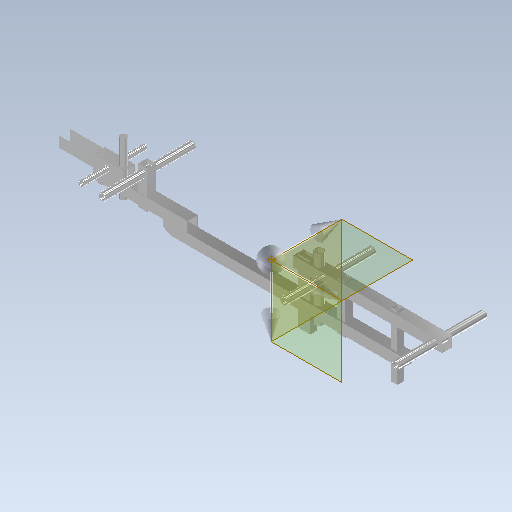
# Autodesk Inventor part: skeleton1
Saved by Autodesk Inventor 2020 (Build 240168000, 168)
## iProperties
Created: 2016-11-12
Part Number: skeleton1
Material: Aluminum 6061
Document SubType Name: Modeling
Designer: jous
Density: 2.7 g/cm^3
Appearance: Aluminum - Flat
Mass: 2970.51 g
Surface Area: 10814.6 cm^2
Volume: 1100.19 cm^3
Author: jous
Autodesk Inventor part; units mm, degrees
ref_plane "YZ Plane" through (0, 0, 0) normal (1, 0, 0) x (0, 1, 0)
ref_plane "XZ Plane" through (0, 0, 0) normal (0, 1, 0) x (-1, 0, 0)
ref_plane "XY Plane" through (0, 0, 0) normal (0, 0, 1) x (1, 0, 0)
sketch "cross" plane through (0, 0, 0) normal (0, 0, 1) x (1, 0, 0)
  line L0 (-20, -20) -> (20, -20)
  line L1 (20, -20) -> (20, 20)
  line L2 (20, 20) -> (-20, 20)
  line L3 (-20, 20) -> (-20, -20)
  line L4 (-20, -20) -> (20, 20) construction
  line L5 (20, -20) -> (-20, 20) construction
  line L6 (-18, -18) -> (18, -18)
  line L7 (18, -18) -> (18, 18)
  line L8 (18, 18) -> (-18, 18)
  line L9 (-18, 18) -> (-18, -18)
  line L10 (-18, -18) -> (18, 18) construction
  line L11 (18, -18) -> (-18, 18) construction
  line L12 (0, 0) -> (-194.342538, 0) construction
  line L13 (-105, -22.5) -> (-60, -22.5)
  line L14 (-60, -22.5) -> (-60, 22.5)
  line L15 (-60, 22.5) -> (-105, 22.5)
  line L16 (-105, 22.5) -> (-105, -22.5)
  line L17 (-105, -22.5) -> (-60, 22.5) construction
  line L18 (-60, -22.5) -> (-105, 22.5) construction
  line L19 (-103, -20.5) -> (-62, -20.5)
  line L20 (-62, -20.5) -> (-62, 20.5)
  line L21 (-62, 20.5) -> (-103, 20.5)
  line L22 (-103, 20.5) -> (-103, -20.5)
  line L23 (-103, -20.5) -> (-62, 20.5) construction
  line L24 (-62, -20.5) -> (-103, 20.5) construction
  line L25 (-105, 22.5) -> (-99, 22.5)
  line L26 (-99, 22.5) -> (-99, -22.5)
  line L27 (-99, -22.5) -> (-105, -22.5)
  line L28 (-105, -22.5) -> (-105, 22.5)
  line L29 (-103, -20.5) -> (-99, -20.5)
  line L30 (-99, -20.5) -> (-99, 20.5)
  line L31 (-99, 20.5) -> (-103, 20.5)
  line L32 (-103, 20.5) -> (-103, -20.5)
  line L33 (-60, 20) -> (-20, 20)
  line L34 (-20, 20) -> (-20, -20)
  line L35 (-20, -20) -> (-60, -20)
  line L36 (-60, -20) -> (-60, 20)
  line L37 (-60, 20) -> (-20, -20) construction
  line L38 (-20, 20) -> (-60, -20) construction
  line L39 (-58, 18) -> (-22, 18)
  line L40 (-22, 18) -> (-22, -18)
  line L41 (-22, -18) -> (-58, -18)
  line L42 (-58, -18) -> (-58, 18)
  line L43 (-58, 18) -> (-22, -18) construction
  line L44 (-22, 18) -> (-58, -18) construction
  point P0 (-82.5, 0)
  point P1 (-40, 0)
  point P2 (-40, 0)
  dimension "d0" = 40
  dimension "d1" = 40
  dimension "d2" = 36
  dimension "d3" = 36
  dimension "d29" = 45
  dimension "d30" = 45
  dimension "d31" = 41
  dimension "d32" = 41
  dimension "d33" = 82.5
  dimension "d167" = 37
  dimension "d172" = 40
  dimension "d173" = 40
  dimension "d174" = 36
  dimension "d175" = 36
  constraints: 90 end point, 16 parallel, 13 midpoint, 9 horizontal, 8 perpendicular, 6 point on line
  measures "d0" distance of L2.end L1.end
  measures "d1" distance of L1.end L0.end
  measures "d2" distance of L8.end L7.end
  measures "d3" distance of L7.end L6.end
  measures "d29" distance of L15.end L14.end
  measures "d30" distance of L14.end L13.end
  measures "d31" distance of L21.end L20.end
  measures "d32" distance of L20.end L19.end
  measures "d33" distance of L12.start point (-82.5, 0)
  measures "d167" distance between parallel lines of L20 L26
  measures "d172" distance of L34.end L35.end
  measures "d173" distance of L33.end L34.end
  measures "d174" distance of L40.end L41.end
  measures "d175" distance of L39.end L40.end
sketch "cross outline for main tube" plane through (0, 0, 0) normal (0, 0, 1) x (1, 0, 0)
  line L0 (-20, 20) -> (-20, -20)
  line L1 (20, 20) -> (-20, 20)
  line L2 (-20, -20) -> (20, -20)
  line L3 (20, -20) -> (20, 20)
  line L4 (-18, 18) -> (-18, -18)
  line L5 (-18, -18) -> (18, -18)
  line L6 (18, -18) -> (18, 18)
  line L7 (18, 18) -> (-18, 18)
extrude "main tube" add sketch "cross outline for main tube" along normal blind 1205.5
sketch "top" plane through (-20, -20, 0) normal (-1, 0, 0) x (0, 0, 1)
  line L0 (0, 40) -> (0, 0) projected
  line L1 (1205.5, 40) -> (1205.5, 0) projected
  line L2 (0, 20) -> (1205.5, 20) construction
  circle A0 centre (40, 20) radius 11.1125
  circle A1 centre (40, 20) radius 12.7
  circle A2 centre (120, 20) radius 10.5
  circle A3 centre (120, 20) radius 12.5
  circle A4 centre (870, 20) radius 16
  circle A5 centre (870, 20) radius 14
  line L3 (802.5, 7.5) -> (847.5, 7.5)
  line L4 (847.5, 7.5) -> (847.5, 32.5)
  line L5 (847.5, 32.5) -> (802.5, 32.5)
  line L6 (802.5, 32.5) -> (802.5, 7.5)
  line L7 (802.5, 7.5) -> (847.5, 32.5) construction
  line L8 (847.5, 7.5) -> (802.5, 32.5) construction
  line L9 (804.5, 9.5) -> (845.5, 9.5)
  line L10 (845.5, 9.5) -> (845.5, 30.5)
  line L11 (845.5, 30.5) -> (804.5, 30.5)
  line L12 (804.5, 30.5) -> (804.5, 9.5)
  line L13 (804.5, 9.5) -> (845.5, 30.5) construction
  line L14 (845.5, 9.5) -> (804.5, 30.5) construction
  line L15 (0, 0) -> (1205.5, 0) projected
  line L16 (0, 40) -> (1205.5, 40) projected
  line L17 (970, 0) -> (970, 40) construction
  line L18 (955, 5) -> (985, 5)
  line L19 (985, 5) -> (985, 35)
  line L20 (985, 35) -> (955, 35)
  line L21 (955, 35) -> (955, 5)
  line L22 (955, 5) -> (985, 35) construction
  line L23 (985, 5) -> (955, 35) construction
  line L24 (957, 7) -> (983, 7)
  line L25 (983, 7) -> (983, 33)
  line L26 (983, 33) -> (957, 33)
  line L27 (957, 33) -> (957, 7)
  line L28 (957, 7) -> (983, 33) construction
  line L29 (983, 7) -> (957, 33) construction
  line L30 (1159.5, 9.5) -> (1180.5, 9.5)
  line L31 (1180.5, 9.5) -> (1180.5, 30.5)
  line L32 (1180.5, 30.5) -> (1159.5, 30.5)
  line L33 (1159.5, 30.5) -> (1159.5, 9.5)
  line L34 (1159.5, 9.5) -> (1180.5, 30.5) construction
  line L35 (1180.5, 9.5) -> (1159.5, 30.5) construction
  line L36 (1157.5, 7.5) -> (1182.5, 7.5)
  line L37 (1182.5, 7.5) -> (1182.5, 32.5)
  line L38 (1182.5, 32.5) -> (1157.5, 32.5)
  line L39 (1157.5, 32.5) -> (1157.5, 7.5)
  line L40 (1157.5, 7.5) -> (1182.5, 32.5) construction
  line L41 (1182.5, 7.5) -> (1157.5, 32.5) construction
  line L42 (192.5, 37.5) -> (227.5, 37.5)
  line L43 (227.5, 37.5) -> (227.5, 2.5)
  line L44 (227.5, 2.5) -> (192.5, 2.5)
  line L45 (192.5, 2.5) -> (192.5, 37.5)
  line L46 (192.5, 37.5) -> (227.5, 2.5) construction
  line L47 (227.5, 37.5) -> (192.5, 2.5) construction
  line L48 (194.5, 4.5) -> (225.5, 4.5)
  line L49 (225.5, 4.5) -> (225.5, 35.5)
  line L50 (225.5, 35.5) -> (194.5, 35.5)
  line L51 (194.5, 35.5) -> (194.5, 4.5)
  line L52 (194.5, 4.5) -> (225.5, 35.5) construction
  line L53 (225.5, 4.5) -> (194.5, 35.5) construction
  point P0 (825, 20)
  point P1 (970, 20)
  point P2 (1170, 20)
  point P3 (210, 20)
  dimension "d38" = 22.225
  dimension "d39" = 40
  dimension "d40" = 25.4
  dimension "d50" = 21
  dimension "d51" = 25
  dimension "d52" = 120
  dimension "d59" = 32
  dimension "d60" = 28
  dimension "d61" = 870
  dimension "d66" = 45
  dimension "d67" = 25
  dimension "d68" = 41
  dimension "d69" = 21
  dimension "d71" = 45
  dimension "d72" = 30
  dimension "d73" = 30
  dimension "d74" = 26
  dimension "d75" = 26
  dimension "d76" = 100
  dimension "d192" = 21
  dimension "d193" = 21
  dimension "d194" = 25
  dimension "d195" = 25
  dimension "d196" = 300
  dimension "d208" = 35
  dimension "d209" = 35
  dimension "d210" = 31
  dimension "d211" = 31
  dimension "d212" = 210
  constraints: 98 end point, 17 midpoint, 16 parallel, 9 perpendicular, 8 horizontal, 6 centre point, 3 coincident, 2 point on line, 10 other
  measures "d38" diameter of A0
  measures "d39" distance from line of A0.centre L0
  measures "d40" diameter of A1
  measures "d50" diameter of A2
  measures "d51" diameter of A3
  measures "d52" distance from line of A3.centre L0
  measures "d59" diameter of A4
  measures "d60" diameter of A5
  measures "d61" distance from line of A4.centre L0
  measures "d66" distance of L5.end L4.end
  measures "d67" distance of L4.end L3.end
  measures "d68" distance of L11.end L10.end
  measures "d69" distance of L10.end L9.end
  measures "d71" distance of A4.centre point (825, 20)
  measures "d72" distance of L20.end L19.end
  measures "d73" distance of L19.end L18.end
  measures "d74" distance of L26.end L25.end
  measures "d75" distance of L25.end L24.end
  measures "d76" distance of point (970, 20) A4.centre
  measures "d192" distance of L32.end L31.end
  measures "d193" distance of L31.end L30.end
  measures "d194" distance of L38.end L37.end
  measures "d195" distance of L37.end L36.end
  measures "d196" distance of point (1170, 20) A4.centre
  measures "d208" distance of L43.end L44.end
  measures "d209" distance of L42.end L43.end
  measures "d210" distance of L50.end L49.end
  measures "d211" distance of L49.end L48.end
  measures "d212" distance from line of L0 point (210, 20)
sketch "cross outline for back tube" plane through (0, 0, 0) normal (0, 0, 1) x (1, 0, 0)
  line L0 (-60, 22.5) -> (-99, 22.5)
  line L1 (-60, -22.5) -> (-60, 22.5)
  line L2 (-99, -22.5) -> (-60, -22.5)
  line L3 (-99, -22.5) -> (-99, -20.5)
  line L4 (-99, -20.5) -> (-62, -20.5)
  line L5 (-62, -20.5) -> (-62, 20.5)
  line L6 (-62, 20.5) -> (-99, 20.5)
  line L7 (-99, 20.5) -> (-99, 22.5)
extrude "back tube" add sketch "cross outline for back tube" along normal blind 140 and the other way blind 105
sketch "cross outline for cut main tube" plane through (0, 0, 0) normal (0, 0, 1) x (1, 0, 0)
  line L0 (-20, 20) -> (-20, -20)
  line L1 (20, 20) -> (-20, 20)
  line L2 (-20, -20) -> (20, -20)
  line L3 (20, -20) -> (20, 20)
  line L4 (-18, 18) -> (-18, -18)
  line L5 (-18, -18) -> (18, -18)
  line L6 (18, -18) -> (18, 18)
  line L7 (18, 18) -> (-18, 18)
extrude "cut main tube" cut sketch "cross outline for cut main tube" along normal blind 290
sketch "top outline for rudder" plane through (-20, -20, 0) normal (-1, 0, 0) x (0, 0, 1)
  circle A0 centre (40, 20) radius 12.7
  circle A1 centre (40, 20) radius 11.1125
extrude "rudder" add sketch "top outline for rudder" along normal blind 92 and the other way blind 13
sketch "top outline for anemo" plane through (-20, -20, 0) normal (-1, 0, 0) x (0, 0, 1)
  circle A0 centre (120, 20) radius 12.5
  circle A1 centre (120, 20) radius 10.5
extrude "anemo" add sketch "top outline for anemo" along normal blind 180 and the other way blind 25
sketch "top outline for sail" plane through (-20, -20, 0) normal (-1, 0, 0) x (0, 0, 1)
  circle A0 centre (870, 20) radius 16
  circle A1 centre (870, 20) radius 14
extrude "sail" add sketch "top outline for sail" along normal blind 175 and the other way blind 65
sketch "top outline for keel/sail vertical" plane through (-20, -20, 0) normal (-1, 0, 0) x (0, 0, 1)
  line L0 (955, 35) -> (955, 5)
  line L1 (985, 35) -> (955, 35)
  line L2 (955, 5) -> (985, 5)
  line L3 (985, 5) -> (985, 35)
  line L4 (957, 33) -> (957, 7)
  line L5 (957, 7) -> (983, 7)
  line L6 (983, 7) -> (983, 33)
  line L7 (983, 33) -> (957, 33)
extrude "keel/sail vertical" add sketch "top outline for keel/sail vertical" along normal blind 134 and the other way blind 50
sketch "Sketch9" plane through (-20, -15, 955) normal (0, 0, -1) x (-1, 0, 0)
  line L0 (0, 0) -> (0, 30) projected
  line L1 (134, 30) -> (134, 0) projected
  line L2 (0, 15) -> (134, 15) construction
  line L3 (89, -5) -> (129, -5)
  line L4 (129, -5) -> (129, 35)
  line L5 (129, 35) -> (89, 35)
  line L6 (89, 35) -> (89, -5)
  line L7 (89, -5) -> (129, 35) construction
  line L8 (129, -5) -> (89, 35) construction
  line L9 (91, -3) -> (127, -3)
  line L10 (127, -3) -> (127, 33)
  line L11 (127, 33) -> (91, 33)
  line L12 (91, 33) -> (91, -3)
  line L13 (91, -3) -> (127, 33) construction
  line L14 (127, -3) -> (91, 33) construction
  point P0 (-20, 15)
  point P1 (109, 15)
  point P2 (109, 15)
  dimension "d110" = 40
  dimension "d111" = 40
  dimension "d112" = 36
  dimension "d113" = 36
  dimension "d226" = 89
  constraints: 26 end point, 7 midpoint, 4 parallel, 2 horizontal, 2 perpendicular, 1 point on line
  measures "d110" distance of L5.end L4.end
  measures "d111" distance of L4.end L3.end
  measures "d112" distance of L11.end L10.end
  measures "d113" distance of L10.end L9.end
  measures "d226" distance between parallel lines of L0 L6
sketch "Sketch9 outline for keel/sail horizontal" plane through (-20, -15, 955) normal (0, 0, -1) x (-1, 0, 0)
  line L0 (89, 35) -> (89, -5)
  line L1 (129, 35) -> (89, 35)
  line L2 (89, -5) -> (129, -5)
  line L3 (129, -5) -> (129, 35)
  line L4 (91, 33) -> (91, -3)
  line L5 (91, -3) -> (127, -3)
  line L6 (127, -3) -> (127, 33)
  line L7 (127, 33) -> (91, 33)
extrude "keel/sail horizontal" add sketch "Sketch9 outline for keel/sail horizontal" along normal blind 165 and the other way blind 405
sketch "cross outline for back tube top" plane through (0, 0, 0) normal (0, 0, 1) x (1, 0, 0)
  line L0 (-105, 22.5) -> (-105, -22.5)
  line L1 (-99, 22.5) -> (-105, 22.5)
  line L2 (-99, 20.5) -> (-99, 22.5)
  line L3 (-99, 20.5) -> (-103, 20.5)
  line L4 (-103, 20.5) -> (-103, -20.5)
  line L5 (-103, -20.5) -> (-99, -20.5)
  line L6 (-99, -22.5) -> (-99, -20.5)
  line L7 (-105, -22.5) -> (-99, -22.5)
extrude "back tube top" add sketch "cross outline for back tube top" along normal blind 140
sketch "cross outline for cut back tube top" plane through (0, 0, 0) normal (0, 0, 1) x (1, 0, 0)
  line L0 (-105, 22.5) -> (-105, -22.5)
  line L1 (-99, 22.5) -> (-105, 22.5)
  line L2 (-99, 20.5) -> (-99, 22.5)
  line L3 (-99, 20.5) -> (-103, 20.5)
  line L4 (-103, 20.5) -> (-103, -20.5)
  line L5 (-103, -20.5) -> (-99, -20.5)
  line L6 (-99, -22.5) -> (-99, -20.5)
  line L7 (-105, -22.5) -> (-99, -22.5)
extrude "cut back tube top" cut sketch "cross outline for cut back tube top" along normal blind 25
sketch "cross outline for middle tube" plane through (0, 0, 0) normal (0, 0, 1) x (1, 0, 0)
  line L0 (-60, -20) -> (-20, -20)
  line L1 (-60, 20) -> (-60, -20)
  line L2 (-20, -20) -> (-20, 20)
  line L3 (-20, 20) -> (-60, 20)
  line L4 (-58, -18) -> (-58, 18)
  line L5 (-22, -18) -> (-58, -18)
  line L6 (-22, 18) -> (-22, -18)
  line L7 (-58, 18) -> (-22, 18)
extrude "middle tube" add sketch "cross outline for middle tube" along normal blind 383.25
sketch "cross outline for cut middle tube" plane through (0, 0, 0) normal (0, 0, 1) x (1, 0, 0)
  line L0 (-60, -20) -> (-20, -20)
  line L1 (-60, 20) -> (-60, -20)
  line L2 (-20, -20) -> (-20, 20)
  line L3 (-20, 20) -> (-60, 20)
  line L4 (-58, -18) -> (-58, 18)
  line L5 (-22, -18) -> (-58, -18)
  line L6 (-22, 18) -> (-22, -18)
  line L7 (-58, 18) -> (-22, 18)
extrude "cut middle tube" cut sketch "cross outline for cut middle tube" along normal blind 21
sketch "Sketch15" plane through (-149, -20, 790) normal (0, -1, 0) x (1, 0, 0)
  circle A0 centre (20, 541) radius 14
  circle A1 centre (20, 541) radius 12
  line L0 (129, -500) -> (129, 415.5)
  line L1 (40, 0) -> (40, 570)
  line L2 (20, 541) -> (20, 114.37273) construction
  circle A2 centre (20, 114.37273) radius 14
  circle A3 centre (20, 114.37273) radius 12
  line L3 (0, 570) -> (40, 570)
  point P0 (149, -790)
  dimension "d150" = 28
  dimension "d151" = 24
  dimension "d200" = 20
  dimension "d201" = 28
  dimension "d202" = 24
  dimension "d203" = 29
  constraints: 4 centre point, 2 coincident, 2 end point, 1 parallel
  measures "d150" diameter of A0
  measures "d151" diameter of A1
  measures "d200" distance from line of L1 A0.centre
  measures "d201" diameter of A2
  measures "d202" diameter of A3
  measures "d203" distance from line of L3 A0.centre
sketch "Sketch15 outline for side tubes 1" plane through (-149, -20, 790) normal (0, -1, 0) x (1, 0, 0)
  circle A0 centre (20, 541) radius 14
  circle A1 centre (20, 541) radius 12
  circle A2 centre (20, 114.37273) radius 14
  circle A3 centre (20, 114.37273) radius 12
extrude "side tubes 1" add sketch "Sketch15 outline for side tubes 1" along normal blind 150 and the other way blind 190
sketch "back side" plane through (-99, -22.5, -105) normal (0, -1, 0) x (1, 0, 0)
  circle A0 centre (16.5, 183.59416) radius 10
  circle A1 centre (16.5, 183.59416) radius 8
  line L0 (39, 0) -> (39, 245)
  point P0 (99, 105)
  dimension "d180" = 20
  dimension "d181" = 16
  dimension "d182" = 22.5
  constraints: 2 centre point, 1 coincident
  measures "d180" diameter of A0
  measures "d181" diameter of A1
  measures "d182" distance from line of L0 A0.centre
sketch "back side outline for side tube 3" plane through (-99, -22.5, -105) normal (0, -1, 0) x (1, 0, 0)
  circle A0 centre (16.5, 183.59416) radius 10
  circle A1 centre (16.5, 183.59416) radius 8
extrude "side tube 3" add sketch "back side outline for side tube 3" along normal blind 100 and the other way blind 145
chamfer "bottom chamfer" distance 15 distance2 30 1 edges at (20, 0, 290)
sketch "top outline for keel tubes" plane through (-20, -20, 0) normal (-1, 0, 0) x (0, 0, 1)
  line L0 (1157.5, 32.5) -> (1157.5, 7.5)
  line L1 (1182.5, 32.5) -> (1157.5, 32.5)
  line L2 (1157.5, 7.5) -> (1182.5, 7.5)
  line L3 (1182.5, 7.5) -> (1182.5, 32.5)
  line L4 (1159.5, 30.5) -> (1159.5, 9.5)
  line L5 (1159.5, 9.5) -> (1180.5, 9.5)
  line L6 (1180.5, 9.5) -> (1180.5, 30.5)
  line L7 (1180.5, 30.5) -> (1159.5, 30.5)
  line L8 (802.5, 32.5) -> (802.5, 7.5)
  line L9 (847.5, 32.5) -> (802.5, 32.5)
  line L10 (802.5, 7.5) -> (847.5, 7.5)
  line L11 (847.5, 7.5) -> (847.5, 32.5)
  line L12 (804.5, 30.5) -> (804.5, 9.5)
  line L13 (804.5, 9.5) -> (845.5, 9.5)
  line L14 (845.5, 9.5) -> (845.5, 30.5)
  line L15 (845.5, 30.5) -> (804.5, 30.5)
extrude "keel tubes" add sketch "top outline for keel tubes" along normal blind 136 and the other way blind 109
sketch "top outline for back vertical" plane through (-20, -20, 0) normal (-1, 0, 0) x (0, 0, 1)
  line L0 (192.5, 37.5) -> (227.5, 37.5)
  line L1 (192.5, 2.5) -> (192.5, 37.5)
  line L2 (227.5, 37.5) -> (227.5, 2.5)
  line L3 (227.5, 2.5) -> (192.5, 2.5)
  line L4 (194.5, 35.5) -> (194.5, 4.5)
  line L5 (194.5, 4.5) -> (225.5, 4.5)
  line L6 (225.5, 4.5) -> (225.5, 35.5)
  line L7 (225.5, 35.5) -> (194.5, 35.5)
extrude "back vertical" add sketch "top outline for back vertical" along normal blind 134 and the other way blind 10
sketch "Sketch17" plane through (-154, -17.5, 227.5) normal (0, -1, 0) x (1, 0, 0)
  line L0 (0, -35) -> (0, 0)
  line L1 (0, 0) -> (94, 0)
  circle A0 centre (25, -17.5) radius 14
  circle A1 centre (25, -17.5) radius 12
  line L2 (0, -35) -> (94, -35)
  line L3 (94, 0) -> (94, -35)
  line L4 (134, -206.5) -> (134, 62.5)
  circle A2 centre (25, 676.87273) radius 12
  line L5 (25, 676.87273) -> (25, -17.5) construction
  line L6 (0, -17.5) -> (101.011933, -17.5) construction
  point P0 (154, -227.5)
  dimension "d217" = 28
  dimension "d218" = 24
  constraints: 4 end point, 2 centre point, 2 coincident, 1 horizontal, 1 midpoint, 1 perpendicular, 1 point on line
  measures "d217" diameter of A0
  measures "d218" diameter of A1
sketch "Sketch17 outline for side tube 2" plane through (-154, -17.5, 227.5) normal (0, -1, 0) x (1, 0, 0)
  circle A0 centre (25, -17.5) radius 14
  circle A1 centre (25, -17.5) radius 12
extrude "side tube 2" add sketch "Sketch17 outline for side tube 2" along normal blind 155 and the other way blind 190
equation "\"d73\" = d72"
equation "\"d75\" = d74"
body "Solid1"
